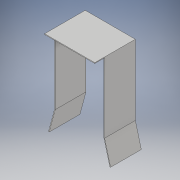
# Autodesk Inventor part: U-Part Gen 2
Saved by Autodesk Inventor 2019 (Build 230136000, 136)
## iProperties
Created: 2019-10-05
Part Number: U-Part Gen 2
Material: Generic
Document SubType Name: Modeling
Designer: Delta
Density: 1 g/cm^3
Appearance: Default
Author: Delta
Autodesk Inventor part; units mm, degrees
ref_plane "YZ Plane" through (0, 0, 0) normal (1, 0, 0) x (0, 1, 0)
ref_plane "XZ Plane" through (0, 0, 0) normal (0, 1, 0) x (-1, 0, 0)
ref_plane "XY Plane" through (0, 0, 0) normal (0, 0, 1) x (1, 0, 0)
sketch "Sketch1" plane through (0, 0, 0) normal (0, 0, 1) x (1, 0, 0)
  line L0 (0, 0) -> (109.855, 0)
  line L1 (109.855, 0) -> (109.855, -1.5875)
  line L2 (109.855, -1.5875) -> (0, -1.5875)
  line L3 (0, -1.5875) -> (0, 0)
  line L4 (109.855, 0) -> (108.2675, 0)
  line L5 (108.2675, 0) -> (108.2675, -154.131)
  line L6 (108.2675, -154.131) -> (109.855, -154.131)
  line L7 (109.855, -154.131) -> (109.855, 0)
  line L8 (0, 0) -> (1.5875, 0)
  line L9 (1.5875, 0) -> (1.5875, -154.131)
  line L10 (1.5875, -154.131) -> (0, -154.131)
  line L11 (0, -154.131) -> (0, 0)
  line L12 (0, -152.5435) -> (25.4, -152.5435) construction
  line L13 (1.5875, -154.131) -> (38.1, -154.131) construction
  line L14 (0, -154.131) -> (-13.0417, -202.8031)
  line L15 (1.5875, -154.131) -> (-11.5605, -203.2)
  line L16 (-13.0417, -202.8031) -> (-11.5605, -203.2)
  line L17 (54.9275, 0) -> (54.9275, -59.745)
  line L18 (109.855, -154.131) -> (122.8967, -202.8031)
  line L19 (108.2675, -154.131) -> (121.4155, -203.2)
  line L20 (122.8967, -202.8031) -> (121.4155, -203.2)
  dimension "d1" = 1.5875
  dimension "d2" = 1.5875
  dimension "d3" = 154.131
  dimension "d5" = 154.131
  dimension "d6" = 1.5875
  dimension "d13" = 1.5875
  dimension "d15" = 106.68
  dimension "d28" = 0
  dimension "d29" = 75
  dimension "d30" = 50.8
  dimension "d31" = 53.34
  dimension "d32" = 203.2
  dimension "d33" = 49.069
  constraints: 42 end point, 6 parallel, 5 horizontal, 4 perpendicular, 2 symmetric about line, 1 midpoint, 1 point on line, 1 vertical
  measures "d1" distance of L0.end L1.end
  measures "d2" distance of L6.end L5.end
  measures "d3" distance of L5.end L4.end
  measures "d5" distance between parallel lines of L10 L0
  measures "d6" distance of L12.start L10.end
  measures "d13" distance between parallel lines of L11 L9
  measures "d15" distance between parallel lines of L5 L9
  measures "d28" angle of L14 L15
  measures "d29" angle of L10 L15
  measures "d30" distance from line of L9.end L16
  measures "d31" distance between parallel lines of L5 L17
  measures "d32" distance from line of L0 L15.end
  measures "d33" distance from line of L10 L15.end
extrude "Extrusion4" add sketch "Sketch1" along normal blind 88.9 contours L0 L9 L2 L3 | L0 L17 L2 L9 | L0 L5 L2 L17 | L0 L1 L2 L5
extrude "Extrusion5" add sketch "Sketch1" along normal blind 67.31 contours L0 L9 L2 L3 | L2 L9 L10 L11 | L10 L15 L16 L14 | L0 L1 L2 L5 | L2 L7 L6 L5 | L6 L18 L20 L19
ref_plane "Work Plane3" through (54.9275, 0, 88.9) normal (1, 0, 0) x (0, 0, -1)
equation "\"d2\" = d1"
equation "\"d3\" = d5"
equation "\"d6\" = d4"
equation "\"d13\" = d2"
equation "\"d4\" = d2"
body "Solid2"
